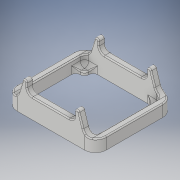
# Autodesk Inventor part: stand
Saved by Autodesk Inventor 2017 (Build 210142000, 142)
## iProperties
Created: 2017-09-15
Part Number: stand
Material: Generic
Document SubType Name: Modeling
Designer: Axel
Density: 1 g/cm^3
Appearance: Default
Author: Axel
Autodesk Inventor part; units mm, degrees
ref_plane "YZ Plane" through (0, 0, 0) normal (1, 0, 0) x (0, 1, 0)
ref_plane "XZ Plane" through (0, 0, 0) normal (0, 1, 0) x (-1, 0, 0)
ref_plane "XY Plane" through (0, 0, 0) normal (0, 0, 1) x (1, 0, 0)
sketch "Sketch1" plane through (0, 0, 0) normal (0, 1, 0) x (-1, 0, 0)
  line L0 (41.0076, 0) -> (35.0076, 0)
  line L1 (35.0076, 0) -> (35.0076, 30)
  line L2 (35.0076, 30) -> (-34.9924, 30)
  line L3 (-34.9924, 30) -> (-34.9924, 0)
  line L4 (-34.9924, 0) -> (-40.9924, 0)
  line L5 (-40.9924, 0) -> (-40.9924, 36)
  line L6 (-40.9924, 36) -> (41.0076, 36)
  line L7 (41.0076, 36) -> (41.0076, 0)
  point P0 (0, 0)
  dimension "d0" = 70
  dimension "d1" = 6
  dimension "d2" = 6
  dimension "d3" = 30
  dimension "d4" = 6
  constraints: 16 end point, 6 perpendicular, 2 point on line, 1 horizontal
  measures "d0" distance between parallel lines of L1 L3
  measures "d1" distance between parallel lines of L7 L1
  measures "d2" distance between parallel lines of L5 L3
  measures "d3" distance between parallel lines of L2 L0
  measures "d4" distance between parallel lines of L6 L2
extrude "Extrusion1" add sketch "Sketch1" along normal blind 30
sketch "Sketch2" plane through (0, 0, 0) normal (0, -1, 0) x (1, 0, 0)
  line L0 (40.9924, 0) -> (40.9924, 36) projected
  line L1 (40.9924, 36) -> (26.9924, 36)
  line L2 (26.9924, 36) -> (26.9924, 22)
  line L3 (26.9924, 22) -> (40.9924, 22)
  line L4 (40.9924, 22) -> (40.9924, 36)
  line L5 (-41.0076, 36) -> (40.9924, 36) projected
  line L6 (-41.0076, 36) -> (-27.0076, 36)
  line L7 (-27.0076, 36) -> (-27.0076, 22)
  line L8 (-27.0076, 22) -> (-41.0076, 22)
  line L9 (-41.0076, 22) -> (-41.0076, 36)
  point P0 (0, 0)
  dimension "d7" = 14
  dimension "d8" = 14
  dimension "d9" = 14
  dimension "d10" = 14
  constraints: 16 end point, 4 parallel, 2 horizontal, 2 perpendicular
  measures "d7" distance of L3.end L2.end
  measures "d8" distance of L2.end L1.end
  measures "d9" distance of L7.end L8.end
  measures "d10" distance of L6.end L7.end
extrude "Extrusion2" add sketch "Sketch2" against normal blind 3
fillet "Fillet1" radius 4 12 edges at (34.9924, 16.5, 30) (26.9924, 1.5, 22) (26.9924, 1.5, 30) (34.9924, 1.5, 22) (30.9924, 3, 30) (34.9924, 3, 26) (-27.0076, 1.5, 30) (-27.0076, 1.5, 22) (-35.0076, 1.5, 22) (-35.0076, 16.5, 30) (-35.0076, 3, 26) (-31.0076, 3, 30)
fillet "Fillet2" radius 1 6 edges at (33.8209, 4.1714, 20.8286) (25.8209, 4.1714, 28.8286) (28.1638, 3, 23.1714) (-25.8362, 4.1714, 28.8286) (-33.8362, 4.1714, 20.8286) (-28.1791, 3, 23.1714)
fillet "Fillet3" radius 10 2 edges at (40.9924, 15, 36) (-41.0076, 15, 36)
sketch "Sketch3" plane through (-31.0076, 0, 36) normal (0, 0, 1) x (1, 0, 0)
  line L0 (72, 11) -> (62, 11)
  line L1 (62, 11) -> (56, 30)
  line L2 (0, 11) -> (6, 30)
  line L3 (-10, 11) -> (0, 11)
  line L4 (6, 30) -> (9, 30)
  line L5 (56, 30) -> (53, 30)
  line L6 (53, 30) -> (53, 18)
  line L7 (9, 30) -> (9, 18)
  line L8 (9, 18) -> (53, 18)
  line L9 (-10, 11) -> (-10, 36)
  line L10 (-10, 36) -> (72, 36)
  line L11 (72, 36) -> (72, 11)
  line L12 (0, 30) -> (62, 30) projected
  point P0 (31.0076, 0)
  point P1 (-10, 0)
  point P2 (72, 0)
  point P3 (31, 18)
  point P4 (31, 30)
  point P5 (31, 30)
  dimension "d16" = 11
  dimension "d17" = 10
  dimension "d18" = 10
  dimension "d19" = 3
  dimension "d20" = 3
  dimension "d21" = 12
  dimension "d22" = 44
  dimension "d23" = 25
  constraints: 24 end point, 5 horizontal alignment, 4 perpendicular, 4 vertical alignment, 2 midpoint, 2 vertical
  measures "d16" distance of point (72, 0) L0.start
  measures "d17" distance of L3.start L2.start
  measures "d18" distance of L0.start L0.end
  measures "d19" distance of L2.end L4.end
  measures "d20" distance of L1.end L5.end
  measures "d21" distance of L5.end L6.end
  measures "d22" distance between parallel lines of L6 L7
  measures "d23" distance between parallel lines of L3 L10
extrude "Extrusion3" cut sketch "Sketch3" against normal blind 100
fillet "Fillet4" radius 7 2 edges at (-31.0076, 11, 33) (30.9924, 11, 33)
fillet "Fillet5" radius 2 4 edges at (-25.0076, 30, 33) (-22.0076, 30, 33) (21.9924, 30, 33) (24.9924, 30, 33)
fillet "Fillet6" radius 5 2 edges at (-22.0076, 18, 33) (21.9924, 18, 33)
mirror "Mirror1" about plane through (0, 0, 0) normal (0, 0, 1)
fillet "Fillet7" radius 1 58 edges at (-33.7957, 11.4035, 28.8685) (-30.088, 14.4787, 30) (-27.6878, 21.5128, 30) (-23.7021, 28.5072, 30) (-22.0076, 24.7658, 30) (-20.5432, 19.4645, 30) (-0.0076, 18, 30) (20.5279, 19.4645, 30) (21.9924, 24.7658, 30) (23.6868, 28.5072, 30) (27.6725, 21.5128, 30) (30.0727, 14.4787, 30) (33.7792, 11.4039, 28.8697) (33.7792, 11.4039, -28.8697) (30.0727, 14.4787, -30) (27.6725, 21.5128, -30) (23.6868, 28.5072, -30) (21.9924, 24.7658, -30) (20.5279, 19.4645, -30) (-0.0076, 18, -30) (-20.5432, 19.4645, -30) (-22.0076, 24.7658, -30) (-23.7021, 28.5072, -30) (-27.6878, 21.5128, -30) (-30.088, 14.4787, -30) (-33.7957, 11.4035, -28.8685) (-39.7054, 11, -30.9345) (-33.3535, 11.5776, -35.7209) (-30.0878, 14.479, -36) (-27.6878, 21.5128, -36) (-23.7021, 28.5072, -36) (-22.0076, 24.7658, -36) (-20.5432, 19.4645, -36) (-0.0076, 18, -36) (20.5279, 19.4645, -36) (21.9924, 24.7658, -36) (23.6868, 28.5072, -36) (27.6725, 21.5128, -36) (30.0725, 14.479, -36) (33.3377, 11.5778, -35.7211) (39.6901, 11, -30.9345) (40.9924, 11, 0) (39.6901, 11, 30.9345) (33.3377, 11.5778, 35.7211) (30.0725, 14.479, 36) (27.6725, 21.5128, 36) (23.6868, 28.5072, 36) (21.9924, 24.7658, 36) (20.5279, 19.4645, 36) (-0.0076, 18, 36) (-20.5432, 19.4645, 36) (-22.0076, 24.7658, 36) (-23.7021, 28.5072, 36) (-27.6878, 21.5128, 36) (-30.0878, 14.479, 36) (-33.3535, 11.5776, 35.7209) (-39.7054, 11, 30.9345) (-41.0076, 11, 0)
body "Solid1"
